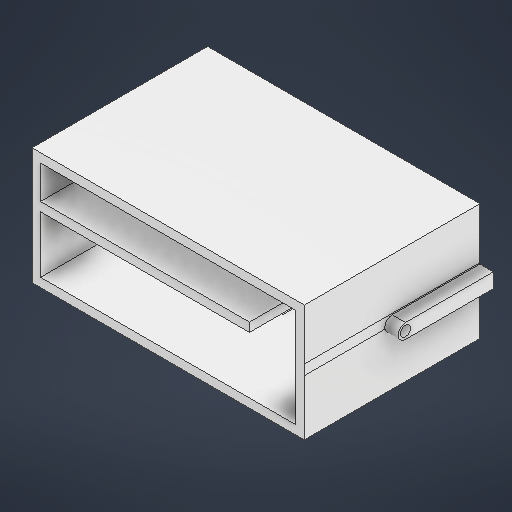
# Autodesk Inventor part: Bakje sensor
Saved by Autodesk Inventor 2026.2 (Build 302298000, 298)
## iProperties
Created: 2026-05-05
Part Number: Bakje sensor
Material: ABS Plastic
Document SubType Name: Modeling
Designer: Gameb
Density: 1.06 g/cm^3
Appearance: Smooth - White
Author: Gameb
Autodesk Inventor part; units mm, degrees
ref_plane "YZ Plane" through (0, 0, 0) normal (1, 0, 0) x (0, 1, 0)
ref_plane "XZ Plane" through (0, 0, 0) normal (0, 1, 0) x (-1, 0, 0)
ref_plane "XY Plane" through (0, 0, 0) normal (0, 0, 1) x (1, 0, 0)
sketch "Sketch1" plane through (0, 0, 0) normal (0, 0, 1) x (1, 0, 0)
  line L0 (16.0355, 8.5355) -> (20.0355, 8.5355)
  line L1 (-73.9645, 8.5355) -> (16.0355, 8.5355)
  line L2 (20.0355, 8.5355) -> (-73.9645, 8.5355)
  line L3 (-73.9645, 27.5374) -> (-73.9645, 23.5355)
  line L4 (40.7522, 23.5355) -> (40.7524, 27.5)
  line L5 (20.0355, 8.5355) -> (20.0355, 12.5391)
  line L6 (40.7522, 12.5355) -> (40.7527, 27.5355)
  line L7 (-73.9639, 27.5391) -> (-73.9643, 12.5391)
  line L8 (-73.9636, 27.541) -> (40.7527, 27.5355)
  line L9 (-73.9643, 12.5391) -> (-73.9636, 27.541)
  line L10 (-77.7958, 27.5374) -> (-77.7958, 31.5374)
  line L11 (-77.7958, 31.5374) -> (-73.7958, 31.5374)
  line L12 (-73.7958, 31.5374) -> (40.9206, 31.5374)
  line L13 (40.9206, 31.5374) -> (44.7523, 31.5374)
  line L14 (44.7523, 27.5355) -> (44.7523, 31.5374)
  line L15 (-77.7958, 27.5374) -> (-77.7958, 8.5355)
  line L16 (-77.7958, 3.9889) -> (-77.7958, 8.5355)
  line L17 (44.7115, 3.9884) -> (44.7523, 8.5718)
  line L18 (-14.4375, 3.9889) -> (-21.9375, 3.9889)
  line L19 (-21.9375, 3.9889) -> (-6.9375, 3.9889)
  line L20 (-6.9375, 3.9889) -> (-6.9375, -15.0111)
  line L21 (-6.9375, -15.0111) -> (-21.9375, -15.0111)
  line L22 (-21.9375, -15.0111) -> (-21.9375, 3.9889)
  line L23 (-23.9375, -15.0111) -> (-23.9375, -17.0111)
  line L24 (-4.9375, -17.0111) -> (-4.9375, 5.9889)
  line L25 (-4.9375, 5.9889) -> (-23.9375, 5.9889)
  line L26 (-23.9375, 5.9889) -> (-23.9375, -17.0111)
  line L27 (-23.9375, -21.0111) -> (-77.7958, -21.0111)
  line L28 (-77.7958, -21.0111) -> (-77.7958, 3.9889)
  line L29 (-73.9645, 8.5355) -> (-73.9645, -17.0111)
  line L30 (-73.9645, -17.0111) -> (-23.9375, -17.0111)
  line L31 (-23.9375, -21.0111) -> (-4.9375, -21.0111)
  line L32 (-4.9375, -21.0111) -> (44.7115, -21.0111)
  line L33 (44.7115, -21.0111) -> (44.7115, 3.9884)
  line L34 (40.7522, 8.5355) -> (40.7522, -17.0111)
  line L35 (40.7522, -17.0111) -> (-4.9375, -17.0111)
  line L36 (-73.9643, 12.5391) -> (20.0355, 12.5391)
  line L37 (-73.9645, 8.5355) -> (20.0355, 8.5355)
  line L38 (40.7522, 12.5355) -> (40.7522, 8.5355)
  line L39 (44.7523, 27.5355) -> (44.7523, 8.5718)
  line L40 (-23.9375, -17.0111) -> (-4.9375, -17.0111)
  point P0 (0, 0)
  point P1 (-73.9645, 27.5355)
  point P2 (40.7521, 27.5)
  constraints: 82 end point, 7 perpendicular, 6 point on line, 5 parallel, 3 vertical, 2 horizontal, 1 collinear
extrude "Extrusion1" add sketch "Sketch1" against normal blind 4 contours L0 L5 L36 L7 L3 L9 L8 L6 L4 L38 L34 L35 L24 L25 L26 L23 L30 L29 L1 | L23 L26 L25 L24 L40 | L10 L11 L12 L13 L14 L39 L17 L33 L32 L31 L27 L28 L16 L15 | L19 L20 L21 L22 L18
extrude "Extrusion2" add sketch "Sketch1" along normal blind 75 contours L10 L11 L12 L13 L14 L39 L17 L33 L32 L31 L27 L28 L16 L15
sketch "Sketch3" plane through (0, 0, 0) normal (0, 0, 1) x (1, 0, 0)
  line L0 (-73.9645, -21.4645) -> (40.7521, -21.4645) projected
  line L1 (40.7521, -21.4645) -> (29.7521, -21.4645)
  line L2 (29.7521, -21.4645) -> (29.7521, -3.4645)
  line L3 (29.7521, -3.4645) -> (40.7521, -3.4645)
  line L4 (40.7521, -3.4645) -> (40.7521, -21.4645)
  circle A0 centre (29.7521, -3.4645) radius 2.5
  point P0 (0, 0)
  dimension "d44" = 11
  dimension "d45" = 18
  dimension "d46" = 5
  constraints: 8 end point, 2 parallel, 1 centre point, 1 coincident, 1 horizontal, 1 perpendicular
  measures "d44" distance of L2.end L3.end
  measures "d45" distance of L1.end L2.end
  measures "d46" diameter of A0
extrude "Extrusion5" cut sketch "Sketch3" against normal blind 4 contours A0 L3 L2 | L2 L3 A0
extrude "Extrusion8" add sketch "Sketch1" along normal blind 35 contours L23 L26 L25 L24 L40
extrude "Extrusion9" add sketch "Sketch1" along normal blind 34 contours L19 L20 L21 L22 L18
sketch "Sketch6" plane through (-73.9645, -17.0111, 75) normal (0, 1, 0) x (1, 0, 0)
  line L0 (69.0269, 40) -> (50.0269, 40) projected
  line L1 (50.0269, 40) -> (69.0269, 40)
  line L2 (69.0269, 75) -> (69.0269, 40) projected
  circle A0 centre (59.5269, 35.25) radius 4.75
  circle A1 centre (59.5269, 35.25) radius 5.75
  point P0 (73.9645, 75)
  dimension "d71" = 11.5
  constraints: 2 centre point, 2 end point, 1 coincident, 1 horizontal
  measures "d71" diameter of A1
extrude "Extrusion10" cut sketch "Sketch6" against normal blind 4 contours A0
extrude "Extrusion11" add sketch "Sketch6" against normal blind 14
sketch "Sketch7" plane through (44.7115, 3.9884, 75) normal (1, -0.0089, 0) x (0, 0, -1)
  line L0 (79, -26.0867) -> (0, -26.0867) projected
  line L1 (79, 26.4598) -> (79, 27.5484) projected
  line L2 (0, -26.0867) -> (79, -26.0867)
  line L3 (79, -26.0867) -> (79, 27.5484)
  line L4 (79, 27.5484) -> (0, 27.5484)
  line L5 (0, 27.5484) -> (0, -26.0867)
  line L6 (0, 0.7308) -> (79, 0.7308)
  line L7 (39.5, -26.0867) -> (39.5, 27.5484)
  circle A0 centre (39.5, 0.7308) radius 2.3
  circle A1 centre (39.5, 0.7308) radius 3.3
  line L8 (39.5, -2.5692) -> (79, -2.5692)
  line L9 (39.5, 4.0308) -> (79, 4.0308)
  point P0 (75, -4.3854)
  dimension "d76" = 4.6
  dimension "d77" = 6.6
  constraints: 16 end point, 5 midpoint, 4 point on line, 3 perpendicular, 2 centre point, 2 parallel, 2 point on circle, 2 tangent, 1 coincident, 1 horizontal
  measures "d76" diameter of A0
  measures "d77" diameter of A1
extrude "Extrusion12" add sketch "Sketch7" along normal blind 6 contours L8 A1 L6 L3 | A1 L6 A0 L7 | L7 A0 L6 A1 | L6 A1 L9 L3 | L6 A0 L7 A1 | A1 L7 A0 L6
sketch "Sketch8" plane through (-77.7958, -21.0111, -4) normal (-1, 0, 0) x (0, 0, 1)
  line L0 (0, 0) -> (79, 0) projected
  line L1 (79, 52.5485) -> (0, 52.5485)
  line L2 (0, 52.5485) -> (0, 0)
  line L3 (0, 0) -> (79, 0)
  line L4 (79, 0) -> (79, 52.5485)
  line L5 (0, 52.5485) -> (79, 52.5485) projected
  line L6 (39.5, 52.5485) -> (39.5, 0)
  line L7 (42.7181, 24.9994) -> (79, 24.9994) projected
  line L8 (79, 24.9994) -> (0, 25.6769)
  line L9 (0, 22.3771) -> (0, 28.9768) projected
  circle A0 centre (39.5, 25.6768) radius 2.3
  ellipse E0 centre (39.5, 25.6769) end of major axis (41.8, 25.6769) minor radius 2.2999 projected
  circle A1 centre (39.5, 25.6768) radius 3.3
  line L10 (39.5, 28.9768) -> (0, 28.9768)
  line L11 (39.5, 22.3768) -> (0, 22.3771)
  point P0 (4, 21.0111)
  dimension "d80" = 6.6
  constraints: 16 end point, 3 midpoint, 3 point on line, 2 centre point, 2 parallel, 2 perpendicular, 2 point on circle, 1 coincident, 1 horizontal, 1 other
  measures "d80" diameter of A1
extrude "Extrusion13" add sketch "Sketch8" along normal blind 6 contours L2 L8 A1 L11 | A1 L8 A0 L6 | L6 A0 L8 A1 | L2 L10 A1 L8 | A1 L6 A0 L8 | L8 A0 L6 A1
body "Solid1"
